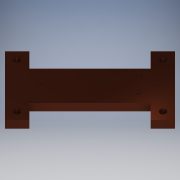
# Autodesk Inventor part: mount-base
Saved by Autodesk Inventor 2017 SP1 (Build 210196100, 196)
## iProperties
Created: 2017-02-03
Part Number: mount-base
Material: Copper
Document SubType Name: Modeling
Designer: Alex
Density: 8.94 g/cm^3
Appearance: Copper - Polished
Author: Alex
Autodesk Inventor part; units mm, degrees
ref_plane "YZ Plane" through (0, 0, 0) normal (1, 0, 0) x (0, 1, 0)
ref_plane "XZ Plane" through (0, 0, 0) normal (0, 1, 0) x (-1, 0, 0)
ref_plane "XY Plane" through (0, 0, 0) normal (0, 0, 1) x (1, 0, 0)
sketch "Sketch1" plane through (0, 0, 0) normal (0, 1, 0) x (-1, 0, 0)
  line L0 (-10, 25) -> (-10, 0)
  line L1 (10, 0) -> (10, 25)
  line L2 (20, 25) -> (10, 25)
  line L3 (-10, 25) -> (-20, 25)
  line L4 (20, 25) -> (20, 35)
  line L5 (-20, 35) -> (-20, 25)
  line L6 (20, 35) -> (-20, 35)
  line L7 (10, 0) -> (-10, 0) construction
  line L8 (20, 30) -> (-20, 30) construction
  line L9 (10, 25) -> (-10, 25) construction
  line L10 (0, 25) -> (0, 0) construction
  line L11 (10, 20) -> (-10, 20) construction
  line L12 (10, 20) -> (0, 20) construction
  line L13 (0, 20) -> (-10, 20) construction
  line L14 (15, 35) -> (15, 30) construction
  line L15 (15, 30) -> (15, 25) construction
  line L16 (-15, 35) -> (-15, 30) construction
  line L17 (-15, 30) -> (-15, 25) construction
  line L18 (-10, -25) -> (-10, 0)
  line L19 (10, 0) -> (10, -25)
  line L20 (20, -25) -> (10, -25)
  line L21 (-10, -25) -> (-20, -25)
  line L22 (20, -25) -> (20, -35)
  line L23 (-20, -35) -> (-20, -25)
  line L24 (20, -35) -> (-20, -35)
  line L25 (20, -30) -> (-20, -30) construction
  line L26 (10, -25) -> (-10, -25) construction
  line L27 (0, -25) -> (0, 0) construction
  line L28 (10, -20) -> (-10, -20) construction
  line L29 (10, -20) -> (0, -20) construction
  line L30 (0, -20) -> (-10, -20) construction
  line L31 (15, -35) -> (15, -30) construction
  line L32 (15, -30) -> (15, -25) construction
  line L33 (-15, -35) -> (-15, -30) construction
  line L34 (-15, -30) -> (-15, -25) construction
  line L35 (0, 20) -> (5, 20) construction
  line L36 (0, 20) -> (-5, 20) construction
  line L37 (0, -20) -> (5, -20) construction
  line L38 (0, -20) -> (-5, -20) construction
  dimension "innerW" = 25
  dimension "d79" = 25
  dimension "outerW" = 10
  dimension "d84" = 5
  dimension "d127" = 20
  constraints: 78 end point, 18 symmetric about line, 13 point on line, 9 midpoint, 3 collinear, 3 perpendicular, 2 parallel, 1 horizontal, 1 vertical
  measures "innerW" distance between parallel lines of L7 L3
  measures "d79" distance between parallel lines of L7 L2
  measures "outerW" distance between parallel lines of L6 L3
  measures "d84" distance between parallel lines of L11 L9
  measures "d127" distance between parallel lines of L0 L1
extrude "Extrusion1" add sketch "Sketch1" along normal blind 5
hole "Hole10" at (-15, 0, 30) at (15, 0, 30) at (15, 0, -30) at (-15, 0, -30) direction (0, 1, 0) diameter 3.4 end through all clearance for "Socket Head Cap Screw ISO 4762" size "M3" standard "ISO"
hole "Hole11" at (0, 0, 20) at (-5, 0, -20) at (5, 0, -20) direction (0, 1, 0) diameter 1.567 end through all thread size "M2x0.4" class "6H" standard "ISO Metric profile"
equation "\"d79\" = innerW"
body "Solid1"
